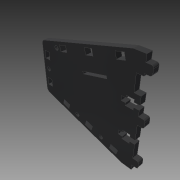
# Autodesk Inventor part: front_panel_2004_brace
Saved by Autodesk Inventor 2014 (Build 180170000, 170)
## iProperties
Created: 2014-01-11
Part Number: front_panel_2004_brace
Material: Generic
Document SubType Name: Modeling
Designer: buben
Density: 1 g/cm^3
Appearance: Anodized - Dark Gray
Author: buben
Autodesk Inventor part; units mm, degrees
ref_plane "YZ Plane" through (0, 0, 0) normal (1, 0, 0) x (0, 1, 0)
ref_plane "XZ Plane" through (0, 0, 0) normal (0, 1, 0) x (-1, 0, 0)
ref_plane "XY Plane" through (0, 0, 0) normal (0, 0, 1) x (1, 0, 0)
sketch "Sketch1" plane through (0, 0, 0) normal (0, 1, 0) x (-1, 0, 0)
  line L0 (0, 108) -> (0, 0)
  line L1 (0, 0) -> (10.412, 0)
  line L2 (10.412, 0) -> (109.1455, 26.4556)
  line L3 (109.1455, 26.4556) -> (109.1455, 81.5444)
  line L4 (109.1455, 81.5444) -> (10.412, 108)
  line L5 (10.412, 108) -> (0, 108)
  line L6 (2.5529, 107) -> (1, 101.2044) construction
  line L7 (1, 101.2044) -> (97.5926, 75.3225) construction
  line L8 (97.5926, 75.3225) -> (99.1455, 81.1181) construction
  line L9 (99.1455, 81.1181) -> (2.5529, 107) construction
  line L10 (1, 6.7956) -> (2.5529, 1) construction
  line L11 (2.5529, 1) -> (99.1455, 26.8819) construction
  line L12 (99.1455, 26.8819) -> (97.5926, 32.6775) construction
  line L13 (97.5926, 32.6775) -> (1, 6.7956) construction
  line L14 (100.1455, 80.5444) -> (106.1455, 80.5444) construction
  line L15 (106.1455, 80.5444) -> (106.1455, 27.4556) construction
  line L16 (106.1455, 27.4556) -> (100.1455, 27.4556) construction
  line L17 (100.1455, 27.4556) -> (100.1455, 80.5444) construction
  line L18 (17.0418, 103.1177) -> (15.4889, 97.3222)
  line L19 (15.4889, 97.3222) -> (23.2163, 95.2516)
  line L20 (23.2163, 95.2516) -> (24.7692, 101.0472)
  line L21 (24.7692, 101.0472) -> (17.0418, 103.1177)
  line L22 (46.9855, 95.0943) -> (45.4326, 89.2988)
  line L23 (45.4326, 89.2988) -> (53.16, 87.2282)
  line L24 (53.16, 87.2282) -> (54.7129, 93.0238)
  line L25 (54.7129, 93.0238) -> (46.9855, 95.0943)
  line L26 (76.9292, 87.0709) -> (75.3763, 81.2754)
  line L27 (75.3763, 81.2754) -> (83.1037, 79.2048)
  line L28 (83.1037, 79.2048) -> (84.6566, 85.0004)
  line L29 (84.6566, 85.0004) -> (76.9292, 87.0709)
  line L30 (15.4889, 10.6778) -> (17.0418, 4.8823)
  line L31 (17.0418, 4.8823) -> (24.7692, 6.9528)
  line L32 (24.7692, 6.9528) -> (23.2163, 12.7484)
  line L33 (23.2163, 12.7484) -> (15.4889, 10.6778)
  line L34 (45.4326, 18.7012) -> (46.9855, 12.9057)
  line L35 (46.9855, 12.9057) -> (54.7129, 14.9762)
  line L36 (54.7129, 14.9762) -> (53.16, 20.7718)
  line L37 (53.16, 20.7718) -> (45.4326, 18.7012)
  line L38 (75.3763, 26.7246) -> (76.9292, 20.9291)
  line L39 (76.9292, 20.9291) -> (84.6566, 22.9996)
  line L40 (84.6566, 22.9996) -> (83.1037, 28.7952)
  line L41 (83.1037, 28.7952) -> (75.3763, 26.7246)
  line L42 (23.9928, 98.1494) -> (46.209, 92.1965) construction
  line L43 (53.9365, 90.126) -> (76.1527, 84.1732) construction
  line L44 (23.9928, 9.8506) -> (46.209, 15.8035) construction
  line L45 (53.9365, 17.874) -> (76.1527, 23.8268) construction
  line L46 (83.8802, 82.1026) -> (98.369, 78.2203) construction
  line L47 (16.2653, 7.7801) -> (1.7765, 3.8978) construction
  line L48 (83.8802, 25.8974) -> (98.369, 29.7797) construction
  line L49 (16.2653, 100.2199) -> (1.7765, 104.1022) construction
  line L50 (100.1455, 72.5444) -> (106.1455, 72.5444)
  line L51 (106.1455, 72.5444) -> (106.1455, 64.5444)
  line L52 (106.1455, 64.5444) -> (100.1455, 64.5444)
  line L53 (100.1455, 64.5444) -> (100.1455, 72.5444)
  line L54 (100.1455, 43.4556) -> (106.1455, 43.4556)
  line L55 (106.1455, 43.4556) -> (106.1455, 35.4556)
  line L56 (106.1455, 35.4556) -> (100.1455, 35.4556)
  line L57 (100.1455, 35.4556) -> (100.1455, 43.4556)
  line L58 (103.1455, 72.5444) -> (103.1455, 80.5444) construction
  line L59 (103.1455, 35.4556) -> (103.1455, 27.4556) construction
  dimension "d0" = 100
  dimension "d1" = 6
  dimension "d3" = 100
  dimension "d4" = 6
  dimension "d7" = 3
  dimension "d8" = 3
  dimension "d9" = 6
  dimension "d10" = 3
  dimension "d11" = 1
  dimension "d12" = 1
  dimension "d13" = 1
  dimension "d14" = 1
  dimension "d15" = 15
  dimension "d16" = 1
  dimension "d17" = 1
  dimension "d18" = 1
  dimension "d19" = 108
  dimension "d20" = 8
  dimension "d21" = 15
  dimension "d22" = 8
  constraints: 120 end point, 25 parallel, 20 midpoint, 19 perpendicular, 16 point on line, 13 equal length, 3 horizontal, 1 vertical, 1 vertical alignment
  measures "d0" distance of L6.end L7.end
  measures "d1" distance of L7.end L8.end
  measures "d3" distance of L12.end L10.start
  measures "d4" distance of L11.end L12.end
  measures "d7" distance between parallel lines of L4 L9
  measures "d8" distance between parallel lines of L2 L11
  measures "d9" distance of L14.start L14.end
  measures "d10" distance between parallel lines of L3 L15
  measures "d11" distance from line of L0 L6.end
  measures "d12" distance from line of L0 L10.start
  measures "d13" distance from line of L6.start L5
  measures "d14" distance from line of L1 L10.end
  measures "d15" angle of L5 L4
  measures "d16" distance from line of L3.end L14
  measures "d17" horizontal distance of L14.start L8.end
  measures "d18" distance from line of L2.end L16
  measures "d19" distance of L0.start L0.end
  measures "d20" distance between parallel lines of L20 L18
  measures "d21" distance of L49.start L49.end
  measures "d22" distance of L59.start L59.end
extrude "Extrusion1" add sketch "Sketch1" along normal blind 6
sketch "Sketch2" plane through (0, 0, 0) normal (0, -1, 0) x (1, 0, 0)
  line L0 (0, 0) -> (0, 108) projected
  line L1 (0, 102) -> (4, 102)
  line L2 (6, 100) -> (6, 96)
  line L3 (4, 94) -> (0, 94)
  line L4 (0, 94) -> (0, 102)
  line L5 (0, 58) -> (4, 58)
  line L6 (6, 56) -> (6, 52)
  line L7 (4, 50) -> (0, 50)
  line L8 (0, 50) -> (0, 58)
  line L9 (0, 14) -> (4, 14)
  line L10 (6, 12) -> (6, 8)
  line L11 (4, 6) -> (0, 6)
  line L12 (0, 6) -> (0, 14)
  arc A0 (6, 100) -> (4, 102) centre (4, 100) ccw
  arc A1 (4, 94) -> (6, 96) centre (4, 96) ccw
  arc A2 (6, 56) -> (4, 58) centre (4, 56) ccw
  arc A3 (4, 50) -> (6, 52) centre (4, 52) ccw
  arc A4 (6, 12) -> (4, 14) centre (4, 12) ccw
  arc A5 (4, 6) -> (6, 8) centre (4, 8) ccw
  line L13 (2, 94) -> (2, 58) construction
  line L14 (2, 50) -> (2, 14) construction
  line L15 (0, 108) -> (-10.412, 108) projected
  point P0 (6, 54)
  point P1 (0, 54)
  dimension "d25" = 2
  dimension "d26" = 6
  dimension "d27" = 8
  dimension "d28" = 8
  dimension "d29" = 8
  dimension "d38" = 6
  constraints: 28 end point, 12 point on circle, 12 tangent, 6 centre point, 6 midpoint, 6 parallel, 5 equal radius, 3 collinear, 3 horizontal, 3 perpendicular, 3 point on line, 1 horizontal alignment
  measures "d25" radius of A0
  measures "d26" distance between parallel lines of L0 L2
  measures "d27" distance between parallel lines of L3 L1
  measures "d28" distance between parallel lines of L7 L5
  measures "d29" distance between parallel lines of L11 L9
  measures "d38" distance between parallel lines of L15 L1
extrude "Extrusion2" add sketch "Sketch2" against normal blind 6
sketch "Sketch3" plane through (0, 0, 0) normal (0, -1, 0) x (1, 0, 0)
  line L0 (0, 58) -> (0, 94) projected
  line L1 (0, 108) -> (-10.412, 108) projected
  line L2 (0, 92) -> (-6, 92)
  line L3 (-6, 92) -> (-6, 76)
  line L4 (-6, 76) -> (0, 76)
  line L5 (0, 76) -> (0, 92)
  dimension "d33" = 16
  dimension "d34" = 6
  dimension "d35" = 16
  constraints: 8 end point, 2 parallel, 1 horizontal, 1 perpendicular, 1 point on line
  measures "d33" distance between parallel lines of L1 L2
  measures "d34" distance of L2.start L2.end
  measures "d35" distance of L2.end L3.end
extrude "Extrusion3" cut sketch "Sketch3" against normal blind 6
sketch "Sketch4" plane through (0, 0, 0) normal (0, -1, 0) x (1, 0, 0)
  line L0 (-10.412, 108) -> (-109.1455, 81.5444) projected
  line L1 (0, 58) -> (0, 76) projected
  line L2 (-23.2163, 95.2516) -> (-24.7692, 101.0472) projected
  line L3 (-56.7165, 71.5226) -> (-56.0695, 69.1077)
  line L4 (-56.0695, 69.1077) -> (-30.9554, 75.837)
  line L5 (-30.9554, 75.837) -> (-31.6024, 78.2519)
  line L6 (-31.6024, 78.2519) -> (-56.7165, 71.5226)
  line L7 (-56.1041, 71.169) -> (-55.7159, 69.7201) construction
  line L8 (-55.7159, 69.7201) -> (-31.5678, 76.1906) construction
  line L9 (-31.5678, 76.1906) -> (-31.956, 77.6395) construction
  line L10 (-31.956, 77.6395) -> (-56.1041, 71.169) construction
  line L11 (-44.1595, 74.8872) -> (-43.5124, 72.4724) construction
  line L12 (-31.2789, 77.0445) -> (-56.393, 70.3152) construction
  point P0 (-44.0301, 74.4042)
  point P1 (-31.7619, 76.915)
  dimension "d39" = 26
  dimension "d41" = 2.5
  dimension "d43" = 1.5
  dimension "d44" = 25
  dimension "d45" = 31.956
  dimension "d48" = 23.75
  constraints: 20 end point, 6 midpoint, 5 parallel, 3 perpendicular, 2 point on line
  measures "d39" distance of L5.end L3.start
  measures "d41" distance of L3.start L3.end
  measures "d43" distance of L7.start L7.end
  measures "d44" distance of L9.end L7.start
  measures "d45" distance from line of L1 L9.end
  measures "d48" distance between parallel lines of L0 L10
extrude "Extrusion4" cut sketch "Sketch4" against normal through all
chamfer "Chamfer1" distance 2 angle 45 2 edges at (-109.1455, 3, 81.5444) (-109.1455, 3, 26.4556)
sketch "Sketch5" plane through (0, 0, 0) normal (0, -1, 0) x (1, 0, 0)
  line L0 (-83.1037, 79.2048) -> (-84.6566, 85.0004) projected
  circle A0 centre (-88.9513, 80.7438) radius 2.25
  line L1 (-88.9513, 80.7438) -> (-83.8802, 82.1026) construction
  line L2 (-106.1455, 64.5444) -> (-100.1455, 43.4556) construction
  line L3 (-106.1455, 43.4556) -> (-100.1455, 64.5444) construction
  line L4 (-75.3763, 26.7246) -> (-54.7129, 14.9762) construction
  line L5 (-53.16, 20.7718) -> (-76.9292, 20.9291) construction
  line L6 (-45.4326, 18.7012) -> (-24.7692, 6.9528) construction
  line L7 (-46.9855, 12.9057) -> (-23.2163, 12.7484) construction
  circle A1 centre (-103.1455, 54) radius 2.25
  circle A2 centre (-65.0446, 20.8504) radius 2.25
  circle A3 centre (-35.1009, 12.827) radius 2.25
  dimension "d52" = 5.25
  dimension "d53" = 4.5
  constraints: 14 end point, 4 centre point, 4 midpoint, 3 equal radius, 2 parallel, 1 perpendicular
  measures "d52" distance of L1.start L1.end
  measures "d53" diameter of A0
extrude "Extrusion5" cut sketch "Sketch5" against normal through all
sketch "Sketch6" plane through (0, 0, 0) normal (0, -1, 0) x (1, 0, 0)
  line L0 (0, 14) -> (0, 50) projected
  line L1 (4, 58) -> (0, 58) projected
  line L2 (0, 58) -> (0, 76) projected
  line L3 (0, 68.25) -> (0, 63.75)
  line L4 (-16.3, 63.75) -> (-16.3, 68.25)
  line L5 (-12.3, 70.75) -> (-5, 70.75)
  line L6 (-5, 61.25) -> (-12.3, 61.25)
  line L7 (-16.3, 68.25) -> (-12.3, 68.25)
  line L8 (-5, 68.25) -> (0, 68.25)
  line L9 (0, 63.75) -> (-5, 63.75)
  line L10 (-12.3, 63.75) -> (-16.3, 63.75)
  line L11 (-12.3, 61.25) -> (-12.3, 63.75)
  line L12 (-12.3, 68.25) -> (-12.3, 70.75)
  line L13 (-5, 70.75) -> (-5, 68.25)
  line L14 (-5, 63.75) -> (-5, 61.25)
  line L15 (0, 34.25) -> (0, 29.75)
  line L16 (-16.3, 29.75) -> (-16.3, 34.25)
  line L17 (-12.3, 36.75) -> (-5, 36.75)
  line L18 (-5, 27.25) -> (-12.3, 27.25)
  line L19 (-16.3, 34.25) -> (-12.3, 34.25)
  line L20 (-5, 34.25) -> (0, 34.25)
  line L21 (0, 29.75) -> (-5, 29.75)
  line L22 (-12.3, 29.75) -> (-16.3, 29.75)
  line L23 (-12.3, 27.25) -> (-12.3, 29.75)
  line L24 (-12.3, 34.25) -> (-12.3, 36.75)
  line L25 (-5, 36.75) -> (-5, 34.25)
  line L26 (-5, 29.75) -> (-5, 27.25)
  point P0 (0, 32)
  point P1 (-16.3, 66)
  dimension "d56" = 4.5
  dimension "d57" = 2.5
  dimension "d58" = 2.5
  dimension "d59" = 4
  dimension "d60" = 5
  dimension "d61" = 7.3
  dimension "d62" = 4.5
  dimension "d63" = 2.5
  dimension "d64" = 2.5
  dimension "d65" = 4
  dimension "d66" = 5
  dimension "d67" = 7.3
  dimension "d68" = 8
  constraints: 48 end point, 20 parallel, 9 collinear, 8 perpendicular, 6 horizontal, 3 midpoint
  measures "d56" distance of L4.start L4.end
  measures "d57" distance of L7.end L5.start
  measures "d58" distance of L6.end L10.start
  measures "d59" distance of L4.end L7.end
  measures "d60" distance of L8.start L3.start
  measures "d61" distance of L5.start L5.end
  measures "d62" distance of L16.start L19.start
  measures "d63" distance of L24.start L17.start
  measures "d64" distance of L23.start L23.end
  measures "d65" distance of L19.start L24.start
  measures "d66" distance of L20.start L15.start
  measures "d67" distance of L17.start L25.start
  measures "d68" distance from line of point (-16.3, 66) L1
extrude "Extrusion6" cut sketch "Sketch6" against normal through all
equation "\"d3\" = d0"
equation "\"d4\" = d1"
equation "\"d8\" = d7"
equation "\"d9\" = d1"
equation "\"d10\" = d7"
equation "\"d12\" = d11"
equation "\"d28\" = d27"
equation "\"d29\" = d28"
equation "\"d58\" = d57"
equation "\"d64\" = d63"
body "Solid1"
